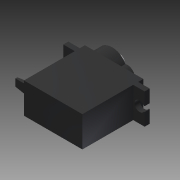
# Autodesk Inventor part: serwo 2.8kg DS939HV
Saved by Autodesk Inventor 2013 (Build 170138000, 138)
## iProperties
Created: 2013-03-06
Part Number: serwo 2.8kg DS939HV
Material: Generic
Document SubType Name: Modeling
Designer: Masta
Density: 2.01644 g/cm^3
Mass: 15 g
Surface Area: 28.4089 cm^2
Volume: 7.43886 cm^3
Author: Masta
Autodesk Inventor part; units mm, degrees
ref_plane "YZ Plane" through (0, 0, 0) normal (1, 0, 0) x (0, 1, 0)
ref_plane "XZ Plane" through (0, 0, 0) normal (0, 1, 0) x (-1, 0, 0)
ref_plane "XY Plane" through (0, 0, 0) normal (0, 0, 1) x (1, 0, 0)
sketch "Sketch1" plane through (0, 0, 0) normal (0, 1, 0) x (-1, 0, 0)
  line L0 (11.5, 6) -> (-11.5, 6)
  line L1 (-11.5, 6) -> (-11.5, -6)
  line L2 (-11.5, -6) -> (11.5, -6)
  line L3 (11.5, -6) -> (11.5, 6)
  line L4 (11.5, 6) -> (-11.5, -6) construction
  line L5 (-11.5, 6) -> (11.5, -6) construction
  line L6 (16, -6) -> (16, -1)
  line L7 (11.5, -6) -> (16, -6)
  line L8 (11.5, 6) -> (16, 6)
  line L9 (-11.5, 6) -> (-16, 6)
  line L10 (-11.5, -6) -> (-16, -6)
  line L11 (-11.5, 0) -> (11.5, 0) construction
  line L12 (0, 6) -> (0, -6) construction
  line L13 (16, -1) -> (15.7321, -1)
  line L14 (16, 1) -> (15.7321, 1)
  circle A0 centre (14, 0) radius 2
  line L15 (-16, 6) -> (-16, -6)
  line L16 (16, 1) -> (16, 6)
  line L17 (16, -1) -> (16, 1)
  line L18 (-16, 6) -> (16, -6) construction
  line L19 (-16, -6) -> (16, 6) construction
  line L20 (14, 0) -> (11.5, 0) construction
  point P0 (0, 0)
  point P1 (0, 0)
  dimension "d0" = 23
  dimension "d1" = 12
  dimension "d2" = 32
  dimension "d40" = 4
  dimension "d41" = 2
  dimension "d42" = 14
  constraints: 42 end point, 7 midpoint, 7 parallel, 5 perpendicular, 2 collinear, 2 point on circle, 1 centre point, 1 coincident, 1 horizontal, 1 other
  measures "d0" distance of L2.end L1.end
  measures "d1" distance of L1.end L0.end
  measures "d2" distance of L10.end L6.start
  measures "d40" diameter of A0
  measures "d41" distance between parallel lines of L14 L13
  measures "d42" distance of point (0, 0) L20.start
extrude "Extrusion1" add sketch "Sketch1" along normal blind 4 and the other way blind 20 contours L3 L2 L1 L0
extrude "Extrusion2" add sketch "Sketch1" along normal blind 2 contours L8 L16 L14 A0 L13 L6 L7 L3
sketch "Sketch2" plane through (0, 4, 0) normal (0, 1, 0) x (1, 0, 0)
  line L0 (-11.5, 6) -> (-11.5, -6) projected
  circle A0 centre (-5.5, 0) radius 6
  line L1 (-5.5, 0) -> (0, 0) construction
  line L2 (11.5, 6) -> (-11.5, 6) projected
  circle A1 centre (0.5, 0) radius 3
  line L3 (0, 0) -> (0.5, 0) construction
  dimension "d14" = 12
  dimension "d15" = 6
  dimension "d43" = 6
  dimension "d44" = 6
  constraints: 4 end point, 2 centre point, 1 parallel, 1 perpendicular
  measures "d14" diameter of A0
  measures "d15" distance from line of L1.start L0
  measures "d43" diameter of A1
  measures "d44" distance of L3.end L1.start
extrude "Extrusion3" add sketch "Sketch2" along normal blind 4.7 contours A0 A1 | A1 A0 | A0 A1
sketch "Sketch3" plane through (-5.5, 8.7, 0) normal (0, 1, 0) x (0, 0, 1)
  circle A0 centre (0, 0) radius 6 projected
  circle A1 centre (0, 0) radius 2.4
  point P0 (0, 5.5)
  dimension "d18" = 4.8
  constraints: 1 centre point, 1 coincident
  measures "d18" diameter of A1
extrude "Extrusion4" add sketch "Sketch3" along normal blind 2.8 contours A1
sketch "Sketch4" plane through (-11.5, -20, -6) normal (-1, 0, 0) x (0, 0, 1)
  line L0 (12, 20) -> (0, 20) projected
  line L1 (4, 3) -> (8, 3)
  line L2 (8, 3) -> (8, 5)
  line L3 (8, 5) -> (4, 5)
  line L4 (4, 5) -> (4, 3)
  line L5 (4, 3) -> (8, 5) construction
  line L6 (8, 3) -> (4, 5) construction
  line L7 (6, 20) -> (6, 4) construction
  dimension "d21" = 4
  dimension "d22" = 2
  dimension "d23" = 15
  constraints: 14 end point, 3 parallel, 2 midpoint, 1 horizontal, 1 perpendicular
  measures "d21" distance of L3.end L2.end
  measures "d22" distance of L2.end L1.end
  measures "d23" distance between parallel lines of L0 L3
extrude "Extrusion5" add sketch "Sketch4" along normal blind 7 draft -5
sketch "Sketch6" plane through (0, 4, 0) normal (0, 1, 0) x (1, 0, 0)
  line L0 (7.663, -5.1534) -> (7.663, 8.9743) construction
  line L1 (7.663, 8.9743) -> (11.2368, 8.9743) construction
  line L2 (11.2368, 8.9743) -> (11.2368, -5.1534) construction
  line L3 (11.2368, -5.1534) -> (7.663, -5.1534) construction
  spline S0 degree 2 poles (8.5234, -3.6865) (8.7492, -3.6865) (9.1125, -3.8695) (9.2141, -4.0232) knots 0 0 0 1 2 2 2
  spline S1 degree 2 poles (9.2141, -4.0232) (9.2929, -4.1487) (9.3463, -4.4066) (9.3463, -4.607) knots 0 0 0 1 2 2 2
  line L4 (9.3463, -4.607) -> (9.3463, -4.9864)
  line L5 (9.3463, -4.9864) -> (7.6978, -4.9864)
  line L6 (7.6978, -4.9864) -> (7.6978, -4.611)
  spline S2 degree 2 poles (7.6978, -4.611) (7.6978, -4.3785) (7.7672, -4.114) (7.8287, -4.0205) knots 0 0 0 1 2 2 2
  spline S3 degree 2 poles (7.8287, -4.0205) (7.9342, -3.8615) (8.2829, -3.6865) (8.5234, -3.6865) knots 0 0 0 1 2 2 2
  spline S4 degree 2 poles (8.5207, -3.9149) (8.331, -3.9149) (8.0625, -4.0405) (7.9863, -4.1648) knots 0 0 0 1 2 2 2
  spline S5 degree 2 poles (7.9863, -4.1648) (7.9342, -4.2529) (7.8875, -4.452) (7.8875, -4.6003) knots 0 0 0 1 2 2 2
  line L7 (7.8875, -4.6003) -> (7.8875, -4.7673)
  line L8 (7.8875, -4.7673) -> (9.1566, -4.7673)
  line L9 (9.1566, -4.7673) -> (9.1566, -4.6003)
  spline S6 degree 2 poles (9.1566, -4.6003) (9.1566, -4.4547) (9.1099, -4.2342) (9.0471, -4.1447) knots 0 0 0 1 2 2 2
  spline S7 degree 2 poles (9.0471, -4.1447) (8.9696, -4.0298) (8.7131, -3.9149) (8.5207, -3.9149) knots 0 0 0 1 2 2 2
  spline S8 degree 2 poles (9.3757, -2.9891) (9.3757, -3.1682) (9.3009, -3.4193) (9.2475, -3.5302) knots 0 0 0 1 2 2 2
  line L10 (9.2475, -3.5302) -> (8.9723, -3.5302)
  line L11 (8.9723, -3.5302) -> (8.9723, -3.5142)
  spline S9 degree 2 poles (8.9723, -3.5142) (9.0738, -3.406) (9.186, -3.1321) (9.186, -3.0052) knots 0 0 0 1 2 2 2
  spline S10 degree 2 poles (9.186, -3.0052) (9.186, -2.8235) (9.0351, -2.6378) (8.9108, -2.6378) knots 0 0 0 1 2 2 2
  spline S11 degree 2 poles (8.9108, -2.6378) (8.812, -2.6378) (8.689, -2.7353) (8.6583, -2.8409) knots 0 0 0 1 2 2 2
  spline S12 degree 2 poles (8.6583, -2.8409) (8.6369, -2.917) (8.6076, -3.0439) (8.5835, -3.1388) knots 0 0 0 1 2 2 2
  spline S13 degree 2 poles (8.5835, -3.1388) (8.5608, -3.2243) (8.4927, -3.3592) (8.4379, -3.4113) knots 0 0 0 1 2 2 2
  spline S14 degree 2 poles (8.4379, -3.4113) (8.3831, -3.4621) (8.2362, -3.5182) (8.14, -3.5182) knots 0 0 0 1 2 2 2
  spline S15 degree 2 poles (8.14, -3.5182) (7.9396, -3.5182) (7.6684, -3.2056) (7.6684, -2.9638) knots 0 0 0 1 2 2 2
  spline S16 degree 2 poles (7.6684, -2.9638) (7.6684, -2.8248) (7.7232, -2.579) (7.7753, -2.4735) knots 0 0 0 1 2 2 2
  line L12 (7.7753, -2.4735) -> (8.0371, -2.4735)
  line L13 (8.0371, -2.4735) -> (8.0371, -2.4895)
  spline S17 degree 2 poles (8.0371, -2.4895) (7.965, -2.5683) (7.8581, -2.8141) (7.8581, -2.9491) knots 0 0 0 1 2 2 2
  spline S18 degree 2 poles (7.8581, -2.9491) (7.8581, -3.1014) (8.001, -3.2897) (8.1173, -3.2897) knots 0 0 0 1 2 2 2
  spline S19 degree 2 poles (8.1173, -3.2897) (8.2215, -3.2897) (8.3457, -3.1788) (8.3738, -3.0746) knots 0 0 0 1 2 2 2
  spline S20 degree 2 poles (8.3738, -3.0746) (8.3925, -3.0052) (8.4406, -2.8034) (8.4606, -2.7366) knots 0 0 0 1 2 2 2
  spline S21 degree 2 poles (8.4606, -2.7366) (8.5127, -2.567) (8.7224, -2.4093) (8.8761, -2.4093) knots 0 0 0 1 2 2 2
  spline S22 degree 2 poles (8.8761, -2.4093) (8.9736, -2.4093) (9.1606, -2.4882) (9.2261, -2.559) knots 0 0 0 1 2 2 2
  spline S23 degree 2 poles (9.2261, -2.559) (9.2982, -2.6378) (9.3757, -2.8382) (9.3757, -2.9891) knots 0 0 0 1 2 2 2
  spline S24 degree 2 poles (8.2335, -2.2784) (8.1066, -2.2784) (7.8955, -2.1956) (7.8193, -2.1235) knots 0 0 0 1 2 2 2
  spline S25 degree 2 poles (7.8193, -2.1235) (7.7459, -2.0553) (7.6644, -1.8563) (7.6644, -1.7547) knots 0 0 0 1 2 2 2
  spline S26 degree 2 poles (7.6644, -1.7547) (7.6644, -1.6412) (7.7405, -1.4568) (7.8127, -1.3887) knots 0 0 0 1 2 2 2
  spline S27 degree 2 poles (7.8127, -1.3887) (7.9035, -1.3032) (8.1974, -1.2097) (8.4232, -1.2097) knots 0 0 0 1 2 2 2
  spline S28 degree 2 poles (8.4232, -1.2097) (8.6276, -1.2097) (8.9936, -1.3018) (9.1152, -1.3914) knots 0 0 0 1 2 2 2
  spline S29 degree 2 poles (9.1152, -1.3914) (9.2435, -1.4862) (9.3784, -1.7534) (9.3784, -1.9484) knots 0 0 0 1 2 2 2
  spline S30 degree 2 poles (9.3784, -1.9484) (9.3784, -1.9925) (9.369, -2.0927) (9.3557, -2.1355) knots 0 0 0 1 2 2 2
  line L14 (9.3557, -2.1355) -> (9.1433, -2.1355)
  line L15 (9.1433, -2.1355) -> (9.1433, -2.1248)
  spline S31 degree 2 poles (9.1433, -2.1248) (9.1593, -2.0967) (9.1873, -1.9792) (9.1873, -1.9191) knots 0 0 0 1 2 2 2
  spline S32 degree 2 poles (9.1873, -1.9191) (9.1873, -1.7026) (8.9015, -1.4555) (8.6369, -1.4381) knots 0 0 0 1 2 2 2
  spline S33 degree 2 poles (8.6369, -1.4381) (8.6971, -1.5263) (8.7518, -1.6866) (8.7518, -1.7815) knots 0 0 0 1 2 2 2
  spline S34 degree 2 poles (8.7518, -1.7815) (8.7518, -1.8723) (8.7118, -2.0233) (8.6543, -2.0994) knots 0 0 0 1 2 2 2
  spline S35 degree 2 poles (8.6543, -2.0994) (8.5862, -2.1876) (8.3791, -2.2784) (8.2335, -2.2784) knots 0 0 0 1 2 2 2
  spline S36 degree 2 poles (8.3738, -1.4328) (8.2068, -1.4328) (7.9957, -1.4942) (7.9382, -1.549) knots 0 0 0 1 2 2 2
  spline S37 degree 2 poles (7.9382, -1.549) (7.8848, -1.5971) (7.8447, -1.6973) (7.8447, -1.7561) knots 0 0 0 1 2 2 2
  spline S38 degree 2 poles (7.8447, -1.7561) (7.8447, -1.8923) (8.0398, -2.054) (8.2241, -2.054) knots 0 0 0 1 2 2 2
  spline S39 degree 2 poles (8.2241, -2.054) (8.3283, -2.054) (8.4633, -2.0005) (8.5114, -1.9418) knots 0 0 0 1 2 2 2
  spline S40 degree 2 poles (8.5114, -1.9418) (8.5461, -1.899) (8.5688, -1.7935) (8.5688, -1.732) knots 0 0 0 1 2 2 2
  spline S41 degree 2 poles (8.5688, -1.732) (8.5688, -1.6612) (8.5194, -1.4982) (8.478, -1.4368) knots 0 0 0 1 2 2 2
  spline S42 degree 2 poles (8.478, -1.4368) (8.4619, -1.4354) (8.4072, -1.4328) (8.3738, -1.4328) knots 0 0 0 1 2 2 2
  spline S43 degree 2 poles (7.8541, -0.5511) (7.8541, -0.6112) (7.8835, -0.7301) (7.9062, -0.7875) knots 0 0 0 1 2 2 2
  spline S44 degree 2 poles (7.9062, -0.7875) (7.9289, -0.8409) (7.977, -0.9198) (7.9984, -0.9505) knots 0 0 0 1 2 2 2
  line L16 (7.9984, -0.9505) -> (7.9984, -0.9639)
  line L17 (7.9984, -0.9639) -> (7.7646, -0.9639)
  spline S45 degree 2 poles (7.7646, -0.9639) (7.7258, -0.8917) (7.663, -0.6446) (7.663, -0.5337) knots 0 0 0 1 2 2 2
  spline S46 degree 2 poles (7.663, -0.5337) (7.663, -0.4215) (7.7085, -0.2545) (7.7566, -0.1863) knots 0 0 0 1 2 2 2
  spline S47 degree 2 poles (7.7566, -0.1863) (7.8087, -0.1142) (7.9596, -0.0394) (8.0612, -0.0394) knots 0 0 0 1 2 2 2
  spline S48 degree 2 poles (8.0612, -0.0394) (8.1974, -0.0394) (8.4032, -0.2184) (8.4299, -0.344) knots 0 0 0 1 2 2 2
  line L18 (8.4299, -0.344) -> (8.4459, -0.344)
  spline S49 degree 2 poles (8.4459, -0.344) (8.4566, -0.2919) (8.5047, -0.173) (8.5528, -0.1222) knots 0 0 0 1 2 2 2
  spline S50 degree 2 poles (8.5528, -0.1222) (8.5995, -0.0714) (8.7492, -0.0073) (8.8574, -0.0073) knots 0 0 0 1 2 2 2
  spline S51 degree 2 poles (8.8574, -0.0073) (8.9683, -0.0073) (9.1566, -0.0835) (9.2288, -0.1529) knots 0 0 0 1 2 2 2
  spline S52 degree 2 poles (9.2288, -0.1529) (9.3036, -0.2251) (9.3811, -0.4295) (9.3811, -0.5591) knots 0 0 0 1 2 2 2
  spline S53 degree 2 poles (9.3811, -0.5591) (9.3811, -0.6833) (9.3209, -0.9265) (9.2795, -1.0093) knots 0 0 0 1 2 2 2
  line L19 (9.2795, -1.0093) -> (9.0457, -1.0093)
  line L20 (9.0457, -1.0093) -> (9.0457, -0.9932)
  spline S54 degree 2 poles (9.0457, -0.9932) (9.0965, -0.9238) (9.19, -0.6887) (9.19, -0.5724) knots 0 0 0 1 2 2 2
  spline S55 degree 2 poles (9.19, -0.5724) (9.19, -0.5043) (9.1473, -0.368) (9.0978, -0.3226) knots 0 0 0 1 2 2 2
  spline S56 degree 2 poles (9.0978, -0.3226) (9.0484, -0.2785) (8.9308, -0.2318) (8.8413, -0.2318) knots 0 0 0 1 2 2 2
  spline S57 degree 2 poles (8.8413, -0.2318) (8.7518, -0.2318) (8.6356, -0.2839) (8.6022, -0.3306) knots 0 0 0 1 2 2 2
  spline S58 degree 2 poles (8.6022, -0.3306) (8.5688, -0.3774) (8.5434, -0.5043) (8.5434, -0.5791) knots 0 0 0 1 2 2 2
  line L21 (8.5434, -0.5791) -> (8.5434, -0.6726)
  line L22 (8.5434, -0.6726) -> (8.3604, -0.6726)
  line L23 (8.3604, -0.6726) -> (8.3604, -0.5991)
  spline S59 degree 2 poles (8.3604, -0.5991) (8.3604, -0.4509) (8.2188, -0.2638) (8.0839, -0.2638) knots 0 0 0 1 2 2 2
  spline S60 degree 2 poles (8.0839, -0.2638) (8.0211, -0.2638) (7.9316, -0.3119) (7.9048, -0.3507) knots 0 0 0 1 2 2 2
  spline S61 degree 2 poles (7.9048, -0.3507) (7.8768, -0.3921) (7.8541, -0.4936) (7.8541, -0.5511) knots 0 0 0 1 2 2 2
  spline S62 degree 2 poles (8.2335, 0.1957) (8.1066, 0.1957) (7.8955, 0.2786) (7.8193, 0.3507) knots 0 0 0 1 2 2 2
  spline S63 degree 2 poles (7.8193, 0.3507) (7.7459, 0.4188) (7.6644, 0.6179) (7.6644, 0.7194) knots 0 0 0 1 2 2 2
  spline S64 degree 2 poles (7.6644, 0.7194) (7.6644, 0.833) (7.7405, 1.0173) (7.8127, 1.0855) knots 0 0 0 1 2 2 2
  spline S65 degree 2 poles (7.8127, 1.0855) (7.9035, 1.171) (8.1974, 1.2645) (8.4232, 1.2645) knots 0 0 0 1 2 2 2
  spline S66 degree 2 poles (8.4232, 1.2645) (8.6276, 1.2645) (8.9936, 1.1723) (9.1152, 1.0828) knots 0 0 0 1 2 2 2
  spline S67 degree 2 poles (9.1152, 1.0828) (9.2435, 0.988) (9.3784, 0.7208) (9.3784, 0.5257) knots 0 0 0 1 2 2 2
  spline S68 degree 2 poles (9.3784, 0.5257) (9.3784, 0.4816) (9.369, 0.3814) (9.3557, 0.3387) knots 0 0 0 1 2 2 2
  line L24 (9.3557, 0.3387) -> (9.1433, 0.3387)
  line L25 (9.1433, 0.3387) -> (9.1433, 0.3494)
  spline S69 degree 2 poles (9.1433, 0.3494) (9.1593, 0.3774) (9.1873, 0.495) (9.1873, 0.5551) knots 0 0 0 1 2 2 2
  spline S70 degree 2 poles (9.1873, 0.5551) (9.1873, 0.7715) (8.9015, 1.0187) (8.6369, 1.036) knots 0 0 0 1 2 2 2
  spline S71 degree 2 poles (8.6369, 1.036) (8.6971, 0.9479) (8.7518, 0.7876) (8.7518, 0.6927) knots 0 0 0 1 2 2 2
  spline S72 degree 2 poles (8.7518, 0.6927) (8.7518, 0.6019) (8.7118, 0.4509) (8.6543, 0.3748) knots 0 0 0 1 2 2 2
  spline S73 degree 2 poles (8.6543, 0.3748) (8.5862, 0.2866) (8.3791, 0.1957) (8.2335, 0.1957) knots 0 0 0 1 2 2 2
  spline S74 degree 2 poles (8.3738, 1.0414) (8.2068, 1.0414) (7.9957, 0.9799) (7.9382, 0.9252) knots 0 0 0 1 2 2 2
  spline S75 degree 2 poles (7.9382, 0.9252) (7.8848, 0.8771) (7.8447, 0.7769) (7.8447, 0.7181) knots 0 0 0 1 2 2 2
  spline S76 degree 2 poles (7.8447, 0.7181) (7.8447, 0.5818) (8.0398, 0.4202) (8.2241, 0.4202) knots 0 0 0 1 2 2 2
  spline S77 degree 2 poles (8.2241, 0.4202) (8.3283, 0.4202) (8.4633, 0.4736) (8.5114, 0.5324) knots 0 0 0 1 2 2 2
  spline S78 degree 2 poles (8.5114, 0.5324) (8.5461, 0.5751) (8.5688, 0.6807) (8.5688, 0.7421) knots 0 0 0 1 2 2 2
  spline S79 degree 2 poles (8.5688, 0.7421) (8.5688, 0.8129) (8.5194, 0.9759) (8.478, 1.0374) knots 0 0 0 1 2 2 2
  spline S80 degree 2 poles (8.478, 1.0374) (8.4619, 1.0387) (8.4072, 1.0414) (8.3738, 1.0414) knots 0 0 0 1 2 2 2
  line L26 (9.3463, 2.722) -> (9.3463, 2.5029)
  line L27 (9.3463, 2.5029) -> (8.5394, 2.5029)
  line L28 (8.5394, 2.5029) -> (8.5394, 1.7441)
  line L29 (8.5394, 1.7441) -> (9.3463, 1.7441)
  line L30 (9.3463, 1.7441) -> (9.3463, 1.525)
  line L31 (9.3463, 1.525) -> (7.6978, 1.525)
  line L32 (7.6978, 1.525) -> (7.6978, 1.7441)
  line L33 (7.6978, 1.7441) -> (8.3444, 1.7441)
  line L34 (8.3444, 1.7441) -> (8.3444, 2.5029)
  line L35 (8.3444, 2.5029) -> (7.6978, 2.5029)
  line L36 (7.6978, 2.5029) -> (7.6978, 2.722)
  line L37 (7.6978, 2.722) -> (9.3463, 2.722)
  line L38 (7.6978, 4.2517) -> (9.3463, 3.6839)
  line L39 (9.3463, 3.6839) -> (9.3463, 3.4474)
  line L40 (9.3463, 3.4474) -> (7.6978, 2.8796)
  line L41 (7.6978, 2.8796) -> (7.6978, 3.1148)
  line L42 (7.6978, 3.1148) -> (9.0671, 3.5717)
  line L43 (9.0671, 3.5717) -> (7.6978, 4.0286)
  line L44 (7.6978, 4.0286) -> (7.6978, 4.2517)
  point P0 (0, 0)
  constraints: 2 other
emboss "Emboss1" sketch "Sketch6" operation cut depth 0.1 direction (0, -1, 0)
hole "Hole1" at (-5.5, 11.5, 0) direction (0, -1, 0) diameter 2.459 depth 8 tip angle 118 thread size "M3x0.5" class "6H" standard "ISO Metric profile"
mirror "Mirror1" about plane through (0, 0, 0) normal (1, 0, 0) of "Extrusion2"
body "Solid1"
